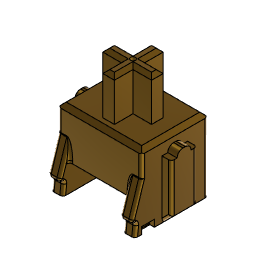
Moyai v22 (Autodesk Fusion 360 design; units mm, degrees)
Autodesk Fusion 360 part; units mm, degrees
note: some values were not read from the file. Set by a fixed rule: which face or edge a step refers to.
sketch "Body" plane through (0, 0, 0) normal (0, 0, 1) x (1, 0, 0) in component "Slider"
  line L0 (0, 0) -> (7.2, 0)
  line L1 (7.2, 0) -> (7.2, 5.7)
  line L2 (7.2, 5.7) -> (0, 5.7)
  line L3 (0, 5.7) -> (0, 0)
  dimension "d4" = 7.2
  dimension "d5" = 5.7
  constraint horizontal L0
  constraint vertical L1
  constraint horizontal L2
  constraint vertical L3
  constraint coincident L0.start L3.end
  measures "d4" distance of L0.start L0.end
  measures "d5" distance of L0.start L2.end
extrude "Extrude1" add sketch "Body" along normal blind 6.3 in component "Slider"
shell "Shell1" thickness 0.44 removed faces 1 at (2.4, 3.8, 0) in component "Slider"
sketch "Inner Thick Stem" plane through (0, 0, 5.86) normal (0, 0, -1) x (1, 0, 0) in component "Slider"
  line L0 (0.44, -0.44) -> (0.44, -5.26)
  line L1 (0.44, -5.26) -> (6.76, -5.26)
  line L2 (6.76, -5.26) -> (6.76, -0.44)
  line L3 (6.76, -0.44) -> (0.44, -0.44)
  line L4 (0.44, -0.44) -> (6.76, -5.26) construction
  line L5 (6.76, -0.44) -> (0.44, -5.26) construction
  circle A0 centre (3.6, -2.85) radius 1.65
  dimension "d12" = 3.3
  constraint coincident L0.start L3.end
  constraint coincident L1.end L2.start
  constraint coincident L2.end L3.start
  constraint coincident L0.end L1.start
  constraint midpoint L5 A0.centre
  measures "d12" diameter of A0
extrude "Extrude2" add sketch "Inner Thick Stem" along normal blind 1.5 contours A0 in component "Slider"
sketch "Inner Spring Stem" plane through (0, 0, 4.36) normal (0, 0, -1) x (1, 0, 0) in component "Slider"
  circle A0 centre (3.6, -2.85) radius 1.65
  circle A1 centre (3.6, -2.85) radius 0.85
  dimension "d16" = 1.7
  constraint concentric A0 A1
  measures "d16" diameter of A1
extrude "Extrude3" add sketch "Inner Spring Stem" along normal blind 4.36 contours A1 in component "Slider"
chamfer "Chamfer1" distance 0.8 angle 45 1 edges at (2.0617, 3.4467, 4.36) in component "Slider"
sketch "Cross" plane through (0, 0, 6.3) normal (0, 0, 1) x (-1, 0, 0) in component "Slider"
  line L0 (0, -5.7) -> (0, 0)
  line L1 (0, 0) -> (-7.2, 0)
  line L2 (-7.2, 0) -> (-7.2, -5.7)
  line L3 (-7.2, -5.7) -> (0, -5.7)
  line L4 (0, -5.7) -> (-7.2, 0) construction
  line L5 (0, 0) -> (-7.2, -5.7) construction
  line L6 (-3.1, -0.75) -> (-4.1, -0.75) construction
  line L7 (-1.5, -2.35) -> (-1.5, -3.35) construction
  line L8 (-4.1, -4.95) -> (-4.1, -3.35)
  line L9 (-4.1, -3.35) -> (-5.7, -3.35)
  line L10 (-5.7, -2.35) -> (-4.1, -2.35)
  line L11 (-4.1, -2.35) -> (-4.1, -0.75)
  line L12 (-4.1, -0.75) -> (-3.1, -0.75)
  line L13 (-3.1, -0.75) -> (-3.1, -2.35)
  line L14 (-3.1, -2.35) -> (-1.5, -2.35)
  line L15 (-1.5, -2.35) -> (-1.5, -3.35)
  line L16 (-1.5, -3.35) -> (-3.1, -3.35)
  line L17 (-3.1, -3.35) -> (-3.1, -4.95)
  line L18 (-3.1, -4.95) -> (-4.1, -4.95)
  line L19 (-5.7, -3.35) -> (-5.7, -2.35)
  dimension "d31" = 1.5
  dimension "d32" = 0.75
  dimension "d35" = 4.2
  dimension "d36" = 4.2
  constraint coincident L0.start L3.end
  constraint coincident L1.end L2.start
  constraint coincident L0.end L1.start
  constraint coincident L2.end L3.start
  constraint horizontal L6
  constraint vertical L7
  constraint perpendicular L8 L18
  constraint perpendicular L10 L19
  measures "d31" distance of L0 L15
  measures "d32" distance of L1 L12
  measures "d35" distance of L7 L19
  measures "d36" distance of L12 L18
extrude "Extrude4" add sketch "Cross" along normal blind 3.6 contours L8 L9 L10 L11 L12 L13 L14 L15 L16 L17 L18 L19 in component "Slider"
chamfer "Chamfer2" distance 0.3 angle 45 12 edges at (2.3, 2.35, 9.9) (1.5, 2.85, 9.9) (2.3, 3.35, 9.9) (3.1, 4.15, 9.9) (3.6, 4.95, 9.9) (4.1, 4.15, 9.9) (4.9, 3.35, 9.9) (5.7, 2.85, 9.9) (4.9, 2.35, 9.9) (4.1, 1.55, 9.9) (3.6, 0.75, 9.9) (3.1, 1.55, 9.9) in component "Slider"
sketch "Wing" plane through (0, 0, 0) normal (-1, 0, 0) x (0, -1, 0) in component "Slider"
  line L0 (-5.7, 0) -> (0, 0)
  line L1 (0, 0) -> (0, 6.3)
  line L2 (0, 6.3) -> (-5.7, 6.3)
  line L3 (-5.7, 6.3) -> (-5.7, 0)
  line L4 (-5.7, 6.3) -> (0, 0) construction
  line L5 (0, 6.3) -> (-5.7, 0) construction
  line L6 (-1.75, 0) -> (-3.95, 0)
  line L7 (-3.95, 0) -> (-3.95, 5.5)
  line L8 (-3.95, 5.5) -> (-1.75, 5.5)
  line L9 (-1.75, 5.5) -> (-1.75, 0)
  line L10 (-1.75, 5.5) -> (-2.25, 5.5)
  line L11 (-2.25, 5.5) -> (-2.25, 5)
  line L12 (-2.25, 5) -> (-1.75, 5)
  line L13 (-1.75, 5) -> (-1.75, 5.5)
  line L14 (-3.95, 5.5) -> (-3.45, 5.5)
  line L15 (-3.45, 5.5) -> (-3.45, 5)
  line L16 (-3.45, 5) -> (-3.95, 5)
  line L17 (-3.95, 5) -> (-3.95, 5.5)
  point P0 (-2.85, 0)
  dimension "d45" = 2.2
  dimension "d46" = 5.5
  dimension "d47" = 1.75
  dimension "d51" = 0.5
  dimension "d52" = 0.5
  dimension "d53" = 0.5
  dimension "d54" = 0.5
  constraint coincident L2.end L3.start
  constraint coincident L0.end L1.start
  constraint coincident L1.end L2.start
  constraint coincident L0.start L3.end
  constraint horizontal L6
  constraint vertical L7
  constraint horizontal L8
  constraint vertical L9
  constraint horizontal L10
  constraint vertical L11
  constraint horizontal L12
  constraint vertical L13
  constraint horizontal L14
  constraint vertical L15
  constraint horizontal L16
  constraint vertical L17
  measures "d45" distance of L6.start L6.end
  measures "d46" distance of L6.start L8.end
  measures "d47" distance of L1 L9
  measures "d51" distance of L8.end L10.end
  measures "d52" distance of L8.end L12.end
  measures "d53" distance of L7.end L14.end
  measures "d54" distance of L7.end L16.end
extrude "Extrude5" add sketch "Wing" along normal blind 0.81 contours L0 L6 L7 L8 L9 L11 L12 L15 L16 in component "Slider"
ref_plane "WorkPlane1" through (3.6, 2.85, 3.15) normal (-1, 0, 0) x (0, -1, 0) in component "Slider"
mirror "Mirror1" about plane through (3.6, 2.85, 3.15) normal (-1, 0, 0) of "Extrude5" in component "Slider"
chamfer "Chamfer3" distance 0.81 angle 45 2 edges at (-0.81, 2.85, 0) (8.01, 2.85, 0) in component "Slider"
extrude "Extrude6" add 1 faces at (6.76, 3.6533, 3.9067) along direction (-1, 0, 0) blind 0.56 in component "Slider"
extrude "Extrude7" add 1 faces at (0.44, 3.6533, 1.9533) along direction (1, 0, 0) blind 0.56 in component "Slider"
sketch "Front and Back Cutouts" plane through (0, 0, 0) normal (0, 0, -1) x (1, 0, 0) in component "Slider"
  line L0 (6.2, -5.26) -> (1, -5.26)
  line L1 (1, -5.26) -> (1, -0.44)
  line L2 (1, -0.44) -> (6.2, -0.44)
  line L3 (6.2, -0.44) -> (6.2, -5.26)
  line L4 (7.2, -3.95) -> (7.2, -1.75)
  line L5 (7.2, -1.75) -> (7.2, 0)
  line L6 (7.2, 0) -> (0, 0)
  line L7 (0, 0) -> (0, -1.75)
  line L8 (0, -1.75) -> (0, -3.95)
  line L9 (0, -3.95) -> (0, -5.7)
  line L10 (0, -5.7) -> (7.2, -5.7)
  line L11 (7.2, -5.7) -> (7.2, -3.95)
  line L12 (1, -0.44) -> (6.2, -0.44)
  line L13 (6.2, -0.44) -> (6.2, 0)
  line L14 (6.2, 0) -> (1, 0)
  line L15 (1, 0) -> (1, -0.44)
  line L16 (1, -5.26) -> (6.2, -5.26)
  line L17 (6.2, -5.26) -> (6.2, -5.7)
  line L18 (6.2, -5.7) -> (1, -5.7)
  line L19 (1, -5.7) -> (1, -5.26)
  dimension "d69" = 5.2
  dimension "d88" = 5.2
  constraint horizontal L12
  constraint vertical L13
  constraint horizontal L14
  constraint vertical L15
  constraint coincident L6 L13.end
  constraint coincident L1.end L2.start
  constraint horizontal L16
  constraint vertical L17
  constraint horizontal L18
  constraint vertical L19
  constraint coincident L10 L17.end
  constraint coincident L0.end L1.start
  measures "d69" distance of L1.end L2.end
  measures "d88" distance of L0.end L0.start
extrude "Extrude8" cut sketch "Front and Back Cutouts" against normal blind 2.3 contours L2 L6 L12 L13 L14 L15 in component "Slider"
extrude "Extrude10" cut sketch "Front and Back Cutouts" against normal blind 1 contours L0 L10 L16 L17 L18 L19 in component "Slider"
sketch "Bump" plane through (0, 0, 0) normal (-1, 0, 0) x (0, -1, 0) in component "Slider"
  line L0 (-1.75, 5) -> (-1.75, 0)
  line L1 (-1.75, 0) -> (0, 0)
  line L2 (0, 0) -> (0, 6.3)
  line L3 (0, 6.3) -> (-5.7, 6.3)
  line L4 (-5.7, 6.3) -> (-5.7, 0)
  line L5 (-5.7, 0) -> (-3.95, 0)
  line L6 (-3.95, 0) -> (-3.95, 5)
  line L7 (-3.95, 5) -> (-3.45, 5)
  line L8 (-3.45, 5) -> (-3.45, 5.5)
  line L9 (-3.45, 5.5) -> (-2.25, 5.5)
  line L10 (-2.25, 5.5) -> (-2.25, 5)
  line L11 (-2.25, 5) -> (-1.75, 5)
  line L12 (0, 6.3) -> (0, 4.1) construction
  line L13 (0, 4.1) -> (0.9, 1.3)
  line L14 (0, 0) -> (3.6, 0) construction
  line L15 (0.9, 1.3) -> (0.5, 1)
  line L16 (0.5, 1) -> (0.6, 0)
  line L17 (0, 0) -> (0.6, 0)
  dimension "d73" = 2.2
  dimension "d74" = 0.9
  dimension "d75" = 1.3
  dimension "d79" = 0.5
  dimension "d82" = 0.3
  dimension "d83" = 0.6
  constraint vertical L12
  constraint coincident L2.end L3.start
  constraint coincident L1.end L2.start
  constraint perpendicular L2 L14
  constraint coincident L14 L16.end
  measures "d73" distance of L2.end L12.end
  measures "d74" distance of L2 L13.end
  measures "d75" distance of L13.end L14
  measures "d79" distance of L2 L15.end
  measures "d82" vertical distance of L13.end L15.end
  measures "d83" distance of L1.end L16.end
extrude "Extrude9" add sketch "Bump" against normal blind 1 contours L2 L13 L15 L16 L17 in component "Slider"
mirror "Mirror2" about plane through (3.6, 2.85, 3.15) normal (-1, 0, 0) of "Extrude9" in component "Slider"
sketch "Leg Cutout" plane through (0, 0, 0) normal (0, 0, -1) x (1, 0, 0) in component "Slider"
  line L0 (6.2, 0.6) -> (6.2, -5.7)
  line L1 (6.2, -5.7) -> (7.2, -5.7)
  line L2 (7.2, -5.7) -> (7.2, -3.95)
  line L3 (7.2, -3.95) -> (7.2, -1.75)
  line L4 (7.2, -1.75) -> (7.2, 0.6)
  line L5 (7.2, 0.6) -> (6.2, 0.6)
  line L6 (6.2, 0) -> (7.2, 0)
  line L7 (7.2, 0) -> (7.2, -1.1)
  line L8 (7.2, -1.1) -> (6.2, -1.1)
  line L9 (6.2, -1.1) -> (6.2, 0)
  point P0 (6.2, 0)
  dimension "d92" = 0.6
  dimension "d94" = 1.1
  constraint horizontal L6
  constraint vertical L7
  constraint horizontal L8
  constraint vertical L9
  constraint coincident L4 L7.end
  constraint coincident P0 L6.start
  measures "d92" distance of L5 L6
  measures "d94" distance of L6.end L7.end
extrude "Extrude11" cut sketch "Leg Cutout" against normal blind 0.6 contours L0 L4 L6 L7 L8 L9 in component "Slider"
sketch "FDM Adhesion Support" plane through (0, 0, 0) normal (0, 0, -1) x (1, 0, 0) in component "Slider"
  line L0 (7.2, -1.1) -> (6.2, -1.1)
  line L1 (6.2, -1.1) -> (6.2, -5.7)
  line L2 (6.2, -5.7) -> (7.2, -5.7)
  line L3 (7.2, -5.7) -> (7.2, -3.95)
  line L4 (7.2, -3.95) -> (7.2, -1.75)
  line L5 (6.59, -1.1) -> (6.81, -1.1)
  line L6 (6.81, -1.1) -> (6.81, 0)
  line L7 (6.81, 0) -> (6.59, 0)
  line L8 (6.59, 0) -> (6.59, -1.1)
  line L9 (7.2, 0) -> (7.2, -1.1)
  line L10 (7.2, -1.75) -> (7.2, -1.1)
  line L11 (7.2, 0.6) -> (6.2, 0.6)
  dimension "d98" = 0.22
  dimension "d99" = 1.1
  dimension "d100" = 0.39
  dimension "d128" = 0.6
  constraint horizontal L5
  constraint vertical L6
  constraint horizontal L7
  constraint vertical L8
  measures "d98" distance of L5.start L5.end
  measures "d99" distance of L5.start L7.end
  measures "d100" distance of L6 L9
  measures "d128" distance of L7 L11
extrude "Extrude12" add sketch "FDM Adhesion Support" against normal blind 0.1 contours L0 L5 L6 L7 L8 in component "Slider"
chamfer "Chamfer4" distance 0.35 angle 45 4 edges at (1, 2.85, 5.86) (3.6, 5.26, 5.86) (6.2, 2.85, 5.86) (3.6, 0.44, 5.86) in component "Slider"
chamfer "Chamfer5" distance 0.35 angle 45 4 edges at (0, 2.85, 6.3) (3.6, 5.7, 6.3) (7.2, 2.85, 6.3) (3.6, 0, 6.3) in component "Slider"
fillet "Fillet1" radius 0.25 4 edges at (0.5, -0.5, 1) (6.7, -0.5, 1) (0.5, -0.9, 1.3) (6.7, -0.9, 1.3) in component "Slider"
fillet "Fillet2" radius 0.25 32 edges at (0, -0.4227, 2.7848) (0, -0.8457, 1.3173) (0, -0.6851, 1.1388) (0, -0.5339, 0.9851) (0, -0.557, 0.4299) (1, -0.4227, 2.7848) (1, -0.8457, 1.3173) (1, -0.6851, 1.1388) (1, -0.5339, 0.9851) (1, -0.557, 0.4299) (6.2, -0.4227, 2.7848) (6.2, -0.8457, 1.3173) (6.2, -0.6851, 1.1388) (6.2, -0.5339, 0.9851) (6.2, -0.557, 0.4299) (7.2, -0.4227, 2.7848) (7.2, -0.8457, 1.3173) (7.2, -0.6851, 1.1388) (7.2, -0.5339, 0.9851) (7.2, -0.557, 0.4299) (7.2, 5.7, 2.975) (7.2, 0, 5.025) (0, 0, 5.025) (0, 5.7, 2.975) (-0.405, 1.75, 0.405) (-0.81, 1.75, 2.905) (-0.405, 3.95, 0.405) (-0.81, 3.95, 2.905) (7.605, 3.95, 0.405) (8.01, 3.95, 2.905) (7.605, 1.75, 0.405) (8.01, 1.75, 2.905) in component "Slider"
fillet "Fillet3" radius 0.5 4 edges at (-0.405, 2.25, 5.5) (-0.405, 3.45, 5.5) (7.605, 3.45, 5.5) (7.605, 2.25, 5.5) in component "Slider"
sketch "Cross Strengthening" plane through (0, 0, 9.9) normal (0, 0, 1) x (-1, 0, 0) in component "Slider"
  line L0 (-3.4, -3.05) -> (-3.8, -2.65) construction
  line L1 (-3.8, -3.05) -> (-3.4, -2.65) construction
  circle A0 centre (-3.6, -2.85) radius 0.22
  line L2 (-5.4, -3.05) -> (-3.8, -3.05)
  line L3 (-3.8, -3.05) -> (-3.8, -4.65)
  line L4 (-3.8, -4.65) -> (-3.4, -4.65)
  line L5 (-3.4, -4.65) -> (-3.4, -3.05)
  line L6 (-3.4, -3.05) -> (-1.8, -3.05)
  line L7 (-1.8, -3.05) -> (-1.8, -2.65)
  line L8 (-1.8, -2.65) -> (-3.4, -2.65)
  line L9 (-3.4, -2.65) -> (-3.4, -1.05)
  line L10 (-3.4, -1.05) -> (-3.8, -1.05)
  line L11 (-3.8, -1.05) -> (-3.8, -2.65)
  line L12 (-3.8, -2.65) -> (-5.4, -2.65)
  line L13 (-5.4, -2.65) -> (-5.4, -3.05)
  dimension "d116" = 0.44
  constraint midpoint L1 A0.centre
  measures "d116" diameter of A0
extrude "Extrude13" cut sketch "Cross Strengthening" against normal blind 5 contours A0 in component "Slider"
fillet "Fillet4" radius 0.25 8 edges at (0.0732, 0.0732, 4.0885) (0.5, 0, 4.1) (0.9268, 0, 3.8607) (1, 0, 2.7915) (7.1268, 0.0732, 4.0885) (6.7, 0, 4.1) (6.2732, 0, 3.8607) (6.2, 0, 2.7915) in component "Slider"
chamfer "Chamfer6" distance 0.35 angle 45 1 edges at (2.8075, 3.1574, 0) in component "Slider"
component "Slider" placed x (1, 0, 0) y (0, 1, 0) z (0, 0, 1) at (0, 0, 0)
equation "body_width = 7.2 mm" comment "Slider body width"
equation "body_depth = 5.7 mm" comment "Slider body depth"
equation "body_height = 6.3 mm" comment "Excluding keycap stem"
equation "d4 = body_width"
equation "d5 = body_depth"
equation "d6 = body_height"
equation "body_walls = 0.44 mm" comment "Recommended max: 0.5mm. Use multiples of extrusion width!"
equation "d9 = body_walls"
equation "spring_thick_dia = 3.3 mm" comment "Outer diameter to grab spring and hold it in place"
equation "spring_thick_height = 1.5 mm" comment "Outer height to grab spring and hold it in place"
equation "d12 = spring_thick_dia"
equation "d13 = spring_thick_height"
equation "spring_stem_dia = 1.7 mm" comment "Inner stem diameter"
equation "d16 = spring_stem_dia"
equation "spring_stem_length = body_height - body_walls - spring_thick_height" comment "Inner stem length"
equation "d18 = spring_stem_length"
equation "spring_stem_transition = ( spring_thick_dia - spring_stem_dia ) / 2" comment "Don't edit! Allows for FDM printing without supports"
equation "d21 = spring_stem_transition"
equation "d31 = cross_width_dist"
equation "d32 = cross_depth_dist"
equation "cross_width_dist = ( body_width / 2 ) - ( cross_width / 2 )" comment "Don't edit! Ensures cross is centered"
equation "cross_depth_dist = ( body_depth / 2 ) - ( cross_depth / 2 )" comment "Don't edit! Ensures cross is centered"
equation "d35 = cross_width"
equation "d36 = cross_depth"
equation "cross_width = 4.2 mm" comment "Cross width (for keycap fitment)"
equation "cross_depth = 4.2 mm" comment "Cross depth (for keycap fitment)"
equation "cross_height = 3.6 mm" comment "Height of cross"
equation "d40 = cross_height"
equation "d42 = cross_chamfer"
equation "cross_chamfer = 0.3 mm" comment "Calculated optimal chamfer for the cross"
equation "d45 = wing_width"
equation "d46 = wing_height"
equation "d47 = wing_offset_center"
equation "wing_offset_center = ( body_depth - wing_width ) / 2" comment "Dont edit! Ensures wings are centered"
equation "wing_width = 2.2 mm" comment "Width of guiding wings"
equation "wing_height = 5.5 mm" comment "Height of guiding wings from the bottom"
equation "d51 = wing_cutout"
equation "d52 = wing_cutout"
equation "d53 = wing_cutout"
equation "d54 = wing_cutout"
equation "wing_cutout = 0.5 mm" comment "Box cutout on the top of the wings"
equation "wing_extrusion = 0.81 mm" comment "Amount of how much the wings poke out"
equation "d57 = wing_extrusion"
equation "d59 = -( body_width / 2 )"
equation "d62 = wing_extrusion"
equation "top_chamfer = 0.35 mm" comment "Amount of internal chamfering"
equation "sides_walls = 1 mm - body_walls" comment "Side reinforcement"
equation "d65 = sides_walls"
equation "d67 = sides_walls"
equation "d69 = ( body_width - 2 mm )"
equation "d70 = -front_cutout_height"
equation "front_cutout_height = 2.3 mm" comment "Leg cutout, necessary for Kailh Pro"
equation "d73 = bump_start_fromtop"
equation "d74 = tactile_bump_outside"
equation "d75 = tactile_bump_frombottom"
equation "tactile_bump_frombottom = 1.3 mm" comment "Distance between bump_start_fromtop and where the tactile bump fully extends in Z direction"
equation "tactile_bump_outside = 0.9 mm" comment "How far the tactile bump goes"
equation "d79 = under_bump_outside"
equation "under_bump_dist = 0.3 mm" comment "Distance between section below the bump and the bump itself in Z direction"
equation "under_bump_outside = 0.5 mm" comment "How far the section below the bump goes"
equation "d82 = under_bump_dist"
equation "d83 = bump_bottom_outside"
equation "d88 = ( body_width - 2 mm )"
equation "back_cutout_height = 1 mm" comment "Back cutout, necessary for Kailh Pro"
equation "d90 = -back_cutout_height"
equation "d92 = bump_bottom_outside"
equation "leg_cutout_length = 1.1 mm" comment "Don't edit! Required cutout on right leg"
equation "d94 = leg_cutout_length"
equation "leg_cutout_depth = 0.6 mm" comment "Don't edit! Required cutout on right leg"
equation "d96 = -leg_cutout_depth"
equation "d98 = body_walls / 2"
equation "d99 = leg_cutout_length"
equation "d100 = 0.5 mm - ( body_walls / 4 )"
equation "d101 = -fdm_adhesion_help"
equation "fdm_adhesion_help = 0.1 mm" comment "Adhesion helper for FDM printers"
equation "d104 = top_chamfer"
equation "d105 = top_chamfer"
equation "general_fillet = 0.25 mm" comment "General filleting of the slider, only edit if needed"
equation "d108 = bump_fillet"
equation "bump_fillet = 0.25 mm" comment "Provides smooth transition for tactile bump, only edit if needed"
equation "d111 = general_fillet"
equation "wing_fillet = wing_cutout" comment "Don't edit! Provides smooth transition for upper portion of the wings"
equation "d114 = wing_fillet"
equation "cross_strength_dia = 0.44 mm" comment "Strengthening bar inside the cross to force more walls in the Slicer"
equation "d116 = cross_strength_dia"
equation "cross_strength_depth = 5 mm" comment "How deep into the Slider does the strengthening bar go?"
equation "d118 = -cross_strength_depth"
equation "bump_start_fromtop = 2.2 mm" comment "Where does the bump start (measured from top, excl. cross)"
equation "bump_bottom_outside = 0.6 mm" comment "How much the pre-bump leg extends from the body"
equation "d128 = bump_bottom_outside"
equation "d130 = general_fillet"
equation "d131 = top_chamfer"
